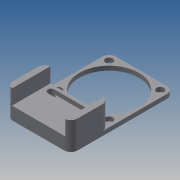
# Autodesk Inventor part: fan zprobe
Saved by Autodesk Inventor 2013 (Build 170138000, 138)
## iProperties
Created: 2017-04-12
Part Number: fan zprobe
Material: Generic
Document SubType Name: Modeling
Designer: employee
Density: 1 g/cm^3
Author: employee
Autodesk Inventor part; units mm, degrees
ref_plane "YZ Plane" through (0, 0, 0) normal (1, 0, 0) x (0, 1, 0)
ref_plane "XZ Plane" through (0, 0, 0) normal (0, 1, 0) x (-1, 0, 0)
ref_plane "XY Plane" through (0, 0, 0) normal (0, 0, 1) x (1, 0, 0)
sketch "Sketch1" plane through (0, 0, 0) normal (0, 0, 1) x (1, 0, 0)
  line L0 (-15.2, 15.2) -> (15.2, 15.2)
  line L1 (15.2, 15.2) -> (15.2, -15.2)
  line L2 (15.2, -15.2) -> (-15.2, -15.2)
  line L3 (-15.2, -15.2) -> (-15.2, 15.2)
  circle A0 centre (0, 0) radius 14
  line L4 (-12, 12) -> (12, 12) construction
  line L5 (12, 12) -> (12, -12) construction
  line L6 (12, -12) -> (-12, -12) construction
  line L7 (-12, -12) -> (-12, 12) construction
  circle A1 centre (-12, 12) radius 1.75
  circle A2 centre (12, 12) radius 1.75
  circle A3 centre (12, -12) radius 1.75
  circle A4 centre (-12, -12) radius 1.75
  dimension "d0" = 30.4
  dimension "d1" = 28
  dimension "d2" = 24
  dimension "d3" = 3.5
  constraints: 16 end point, 7 coincident, 5 centre point, 3 equal radius, 2 horizontal, 18 other
  measures "d0" distance of L2.end L0.start
  measures "d1" diameter of A0
  measures "d2" distance of L6.end L4.start
  measures "d3" diameter of A4
extrude "Extrusion1" add sketch "Sketch1" along normal blind 6
sketch "Sketch2" plane through (0, 0, 6) normal (0, 0, 1) x (1, 0, 0)
  line L0 (-15.2, -15.2) -> (15.2, -15.2) projected
  line L1 (-12.5, -15.2) -> (12.5, -15.2)
  line L2 (12.5, -15.2) -> (12.5, -33.2)
  line L3 (12.5, -33.2) -> (-12.5, -33.2)
  line L4 (-12.5, -33.2) -> (-12.5, -15.2)
  point P0 (0, -15.2)
  dimension "d6" = 25
  dimension "d8" = 18
  constraints: 8 end point, 2 midpoint, 2 parallel, 1 horizontal, 1 perpendicular
  measures "d6" distance of L2.end L3.end
  measures "d8" distance of L1.end L2.end
extrude "Extrusion2" add sketch "Sketch2" against normal up to surface (6 mm away)
sketch "Sketch3" plane through (0, 0, 6) normal (0, 0, 1) x (1, 0, 0)
  circle A0 centre (0, 0) radius 14 projected
  line L0 (-15.2, -15.2) -> (-12.5, -15.2) projected
  line L1 (15.2, -15.2) -> (15.2, 15.2) projected
  line L2 (-9.125, -18.2) -> (9.125, -18.2)
  circle A1 centre (-9.125, -18.2) radius 1.55
  circle A2 centre (9.125, -18.2) radius 1.55
  point P0 (0, -18.2)
  dimension "d11" = 3
  dimension "d12" = 18.25
  dimension "d13" = 3.1
  constraints: 2 centre point, 2 coincident, 2 end point, 1 equal radius, 1 midpoint, 1 perpendicular, 1 vertical alignment
  measures "d11" distance between parallel lines of L0 L2
  measures "d12" distance of L2.start L2.end
  measures "d13" diameter of A2
extrude "Extrusion3" cut sketch "Sketch3" against normal blind 6 contours A1 | A2
sketch "Sketch4" plane through (0, 0, 6) normal (0, 0, 1) x (1, 0, 0)
  circle A0 centre (-9.125, -18.2) radius 1.55 projected
  circle A1 centre (9.125, -18.2) radius 1.55 projected
  line L0 (-9.125, -16.65) -> (9.125, -16.65)
  line L1 (9.125, -19.75) -> (-9.125, -19.75)
  constraints: 4 end point, 4 point on circle, 4 tangent
extrude "Extrusion4" cut sketch "Sketch4" against normal blind 2 contours A0 L0 A1 L1
sketch "Sketch5" plane through (0, 0, 6) normal (0, 0, 1) x (1, 0, 0)
  line L0 (-12.5, -33.2) -> (12.5, -33.2) projected
  line L1 (15.2, -15.2) -> (15.2, 15.2) projected
  line L2 (-15.2, -15.2) -> (-12.5, -15.2)
  line L3 (-12.5, -15.2) -> (-12.5, -33.2)
  line L4 (-12.5, -33.2) -> (-15.2, -33.2)
  line L5 (-15.2, -33.2) -> (-15.2, -15.2)
  line L6 (12.5, -15.2) -> (15.2, -15.2)
  line L7 (15.2, -15.2) -> (15.2, -33.2)
  line L8 (15.2, -33.2) -> (12.5, -33.2)
  line L9 (12.5, -33.2) -> (12.5, -15.2)
  constraints: 16 end point, 4 parallel, 2 horizontal, 2 perpendicular, 2 point on line
extrude "Extrusion5" add sketch "Sketch5" along normal blind 7
sketch "Sketch6" plane through (0, 0, 6) normal (0, 0, -1) x (-1, 0, 0)
  line L0 (15.2, -15.2) -> (15.2, -33.2) projected
  line L1 (15.2, -15.2) -> (12.5, -15.2) projected
  line L2 (12.5, -15.2) -> (12.5, -33.2) projected
  line L3 (15.2, -33.2) -> (12.5, -33.2) projected
  line L4 (-12.5, -15.2) -> (-15.2, -15.2) projected
  line L5 (-15.2, -33.2) -> (-15.2, -15.2) projected
  line L6 (-12.5, -33.2) -> (-15.2, -33.2) projected
  line L7 (-12.5, -33.2) -> (-12.5, -15.2) projected
  point P0 (0, 0)
extrude "Extrusion6" add sketch "Sketch6" along normal up to surface (6 mm away)
fillet "Fillet3" radius 3.2 6 edges at (-15.2, -33.2, 6.5) (15.2, -33.2, 6.5) (15.2, 15.2, 3) (-15.2, 15.2, 3) (15.2, -15.2, 9.5) (-15.2, -15.2, 9.5)
sketch "Sketch7" plane through (0, 0, 6) normal (0, 0, 1) x (1, 0, 0)
  circle A0 centre (0, 0) radius 14 projected
  circle A1 centre (-12, -12) radius 1.75 projected
  circle A2 centre (12, -12) radius 1.75 projected
  circle A3 centre (12, 12) radius 1.75 projected
  circle A4 centre (-12, 12) radius 1.75 projected
  arc A5 (-12, 15.2) -> (-15.2, 12) centre (-12, 12) ccw projected
  line L0 (-15.2, 12) -> (-15.2, -18.3607) projected
  arc A6 (-12.5, -15.2) -> (-15.2, -18.3607) centre (-12, -18.3607) ccw projected
  line L1 (-12.5, -15.2) -> (-12.5, -33.1607) projected
  arc A7 (15.2, -18.3607) -> (12.5, -15.2) centre (12, -18.3607) ccw projected
  line L2 (15.2, -18.3607) -> (15.2, 12) projected
  arc A8 (15.2, 12) -> (12, 15.2) centre (12, 12) ccw projected
  line L3 (12, 15.2) -> (-12, 15.2) projected
  arc A9 (-12, -15.1607) -> (-12.5, -15.2) centre (-12, -18.3607) ccw
  line L4 (-12, -15.1607) -> (12, -15.1607)
  arc A10 (12.5, -15.2) -> (12, -15.1607) centre (12, -18.3607) ccw
  arc A11 (-12.5, -15.2) -> (-15.2, -18.3607) centre (-12, -18.3607) ccw projected
  constraints: 4 point on circle, 3 tangent, 2 centre point, 2 concentric, 2 end point, 1 perpendicular
extrude "Extrusion7" cut sketch "Sketch7" against normal blind 4
body "Solid1"
